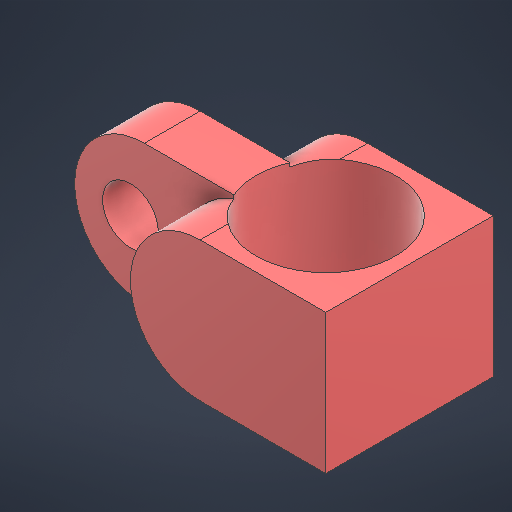
# Autodesk Inventor part: Knee
Saved by Autodesk Inventor 2027 (Build 310192060, 192F)
## iProperties
Created: 2026-08-01
Part Number: Knee
Material: Ogólny
Document SubType Name: Modeling
Designer: User
Density: 1 g/cm^3
Appearance: Domyślna
Author: User
Autodesk Inventor part; units mm, degrees
ref_plane "YZ Plane" through (0, 0, 0) normal (1, 0, 0) x (0, 1, 0)
ref_plane "XZ Plane" through (0, 0, 0) normal (0, 1, 0) x (-1, 0, 0)
ref_plane "XY Plane" through (0, 0, 0) normal (0, 0, 1) x (1, 0, 0)
sketch "Szkic2" plane through (0, 0, 0) normal (0, 1, 0) x (-1, 0, 0)
  line L0 (-11, 6) -> (11, 6)
  line L1 (11, 6) -> (11, -6)
  line L2 (11, -6) -> (-11, -6)
  line L3 (-11, -6) -> (-11, 6)
  line L4 (-11, 6) -> (11, -6) construction
  line L5 (11, 6) -> (-11, -6) construction
  line L6 (-11, 0) -> (-5, 0)
  circle A0 centre (-5, 0) radius 5
  line L7 (11, 0) -> (11, 2)
  line L8 (11, 2) -> (3, 2)
  line L9 (3, 2) -> (3, 6)
  line L10 (11, -6) -> (11, 6)
  line L11 (11, -2) -> (3, -2)
  line L12 (3, -2) -> (3, -6)
  point P0 (0, 0)
  point P1 (3, -6)
  point P2 (11, -2)
  dimension "d11" = 22
  dimension "d12" = 12
  dimension "d13" = 6
  dimension "d14" = 10
  dimension "d15" = 2
  dimension "d16" = 8
  constraints: 26 end point, 5 symmetric about line, 4 midpoint, 3 perpendicular, 3 point on line, 2 horizontal, 2 parallel, 1 centre point, 1 coincident
  measures "d11" distance of L1.end L2.end
  measures "d12" distance of L0.end L1.end
  measures "d13" distance of L6.start L6.end
  measures "d14" diameter of A0
  measures "d15" distance of L7.start L7.end
  measures "d16" distance of L7.end L8.end
extrude "Wyciągnięcie proste3" add sketch "Szkic2" along normal blind 10 contours L0 L9 L8 L1 L11 L12 L2 L3
sketch "Szkic3" plane through (-11, 0, 2) normal (0, 0, 1) x (1, 0, 0)
  line L0 (0, 0) -> (0, 10) projected
  line L1 (8, 0) -> (0, 0) projected
  line L2 (0, 10) -> (0, 0)
  line L3 (8, 0) -> (8, 10) projected
  circle A0 centre (4, 5) radius 2
  point P0 (11, 0)
  dimension "d19" = 4
  dimension "d23" = 4
  constraints: 2 end point, 1 centre point, 1 perpendicular
  measures "d19" diameter of A0
  measures "d23" distance from line of L3 A0.centre
extrude "Wyciągnięcie proste4" cut sketch "Szkic3" against normal blind 32.75
fillet "Zaokrąglenie1" radius 5 6 edges at (-11, 0, 0) (-11, 10, 0) (-3, 0, 4) (-3, 10, 4) (-3, 0, -4) (-3, 10, -4)
